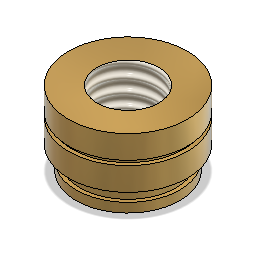
Casting_Plug v3 (Autodesk Fusion 360 archive; units mm, degrees)
design "M4 insert"
Autodesk Fusion 360 part; units mm, degrees
sketch "Sketch1" plane through (0, 0, 0) normal (0, 0, 1) x (1, 0, 0)
  line L0 (2, 0) -> (2.8, 0)
  line L1 (2.8, 0) -> (2.8, 0.5)
  line L2 (2.8, 0.5) -> (2.6, 0.5)
  line L3 (2.6, 0.5) -> (2.6, 1.25)
  line L4 (2.6, 1.25) -> (3.2, 1.25)
  line L5 (3.2, 4) -> (2, 4)
  line L6 (2, 4) -> (2, 0)
  line L7 (3.2, 2.75) -> (3, 2.75)
  line L8 (3, 2.75) -> (3, 2.5)
  line L9 (3, 2.5) -> (3.2, 2.5)
  line L10 (3.2, 1.25) -> (3.2, 2.5)
  line L11 (3.2, 2.75) -> (3.2, 4)
  dimension "d1" = 4
  dimension "d6" = 2
  dimension "d7" = 2.8
  dimension "d8" = 3.2
  dimension "d9" = 2.75
  dimension "d10" = 0.5
  dimension "d11" = 0.25
  dimension "d12" = 0.2
  dimension "d13" = 0.2
  constraint horizontal L0
  constraint perpendicular L0 L1
  constraint perpendicular L1 L2
  constraint perpendicular L2 L3
  constraint perpendicular L3 L4
  constraint perpendicular L4 L10
  constraint perpendicular L5 L10
  constraint perpendicular L0 L6
  constraint coincident L0.start L6
  constraint coincident L0.start L6.end
  constraint horizontal origin L0.start
  constraint coincident L7.start L10
  constraint perpendicular L7 L10
  constraint perpendicular L7 L8
  constraint perpendicular L9 L10
  constraint collinear L10 L11
  constraint equal L10 L11
  measures "d1" distance of L5.end L0.start
  measures "d6" distance of origin L6
  measures "d7" distance of origin L1
  measures "d8" distance of origin L10
  measures "d9" distance of L4.end L5.start
  measures "d10" distance of L0.end L1.end
  measures "d11" distance of L7.end L8.end
  measures "d12" distance of L7.start L7.end
  measures "d13" distance of L1.end L2.end
revolve "Revolve1" add sketch "Sketch1" angle 360 about axis through (0, 1.75, 0) along (0, 1, 0)
thread "Thread1" "ISO Metric profile 4.0 M4x0.7 6H" major diameter 4.1095 minor diameter 3.332 pitch 0.7 angle 60 resizes the face on face at (1.9975, 1.3333, 0.0997)
equation "d7 = ( 5.6 / 2 ) * 1 mm"
equation "d8 = ( 6.4 / 2 ) * 1 mm"
